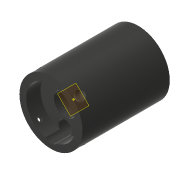
# Autodesk Inventor part: Backshellv1
Saved by Autodesk Inventor 2019.4 (Build 234330000, 330)
## iProperties
Created: 2020-03-14
Part Number: Backshellv1
Material: UHMW, Black
Document SubType Name: Modeling
Designer: Peter
Density: 0.94 g/cm^3
Appearance: Smooth - Black
Mass: 267.904 g
Surface Area: 536.934 cm^2
Volume: 285.004 cm^3
Author: Peter
Autodesk Inventor part; units mm, degrees
ref_plane "YZ Plane" through (0, 0, 0) normal (1, 0, 0) x (0, 1, 0)
ref_plane "XZ Plane" through (0, 0, 0) normal (0, 1, 0) x (-1, 0, 0)
ref_plane "XY Plane" through (0, 0, 0) normal (0, 0, 1) x (1, 0, 0)
sketch "Sketch1" plane through (0, 0, 0) normal (0, 0, 1) x (1, 0, 0)
  circle A0 centre (0, 0) radius 37.5
  dimension "d0" = 75
  constraints: 1 centre point, 1 coincident
  measures "d0" diameter of A0
extrude "Extrusion1" add sketch "Sketch1" along normal blind 104
sketch "Sketch3" plane through (0, 0, 0) normal (0, 0, -1) x (-1, 0, 0)
  circle A0 centre (0, 0) radius 35
  dimension "d6" = 70
  constraints: 1 centre point, 1 coincident
  measures "d6" diameter of A0
extrude "Extrusion3" cut sketch "Sketch3" against normal blind 16.5
sketch "Sketch4" plane through (0, 0, 16.5) normal (0, 0, -1) x (-1, 0, 0)
  circle A0 centre (0, 0) radius 8
  dimension "d9" = 16
  constraints: 1 centre point, 1 coincident
  measures "d9" diameter of A0
extrude "Extrusion4" add sketch "Sketch4" along normal blind 10.5
sketch "Sketch6" plane through (0, 0, 104) normal (0, 0, 1) x (1, 0, 0)
  circle A0 centre (0, 0) radius 16.9805
  constraints: 1 centre point, 1 coincident
hole "Hole1" at (0, 0, 104) direction (0, 0, -1) diameter 27 depth 70 tip angle 118 counterbore diameter 59 counterbore depth 17
sketch "Sketch7" plane through (0, 0, 6) normal (0, 0, -1) x (-1, 0, 0)
  circle A0 centre (0, 0) radius 2.5875
  constraints: 1 centre point, 1 coincident
hole "Hole2" at (0, 0, 6) direction (0, 0, 1) diameter 10.106 end through all thread size "M12x1.75" class "6H" standard "ISO Metric profile"
sketch "Sketch8" plane through (0, 0, 16.5) normal (0, 0, -1) x (-1, 0, 0)
  circle A0 centre (0, 0) radius 24 construction
  circle A1 centre (0, -24) radius 8
  circle A2 centre (0, 24) radius 8
  dimension "d26" = 48
  dimension "d27" = 16
  dimension "d28" = 16
  constraints: 3 centre point, 2 point on circle, 1 coincident
  measures "d26" diameter of A0
  measures "d27" diameter of A2
  measures "d28" diameter of A1
extrude "Extrusion5" cut sketch "Sketch8" against normal through all
sketch "Sketch9" plane through (0, 0, 16.5) normal (0, 0, -1) x (-1, 0, 0)
  circle A0 centre (0, 0) radius 13
  line L0 (0, 0) -> (9.1924, 9.1924)
  line L1 (0, 0) -> (13, 0) construction
  circle A1 centre (9.1924, 9.1924) radius 2.3283
  dimension "d31" = 26
  dimension "d33" = 13
  dimension "d34" = 45
  constraints: 4 end point, 2 centre point, 2 coincident, 1 equal length, 1 horizontal
  measures "d31" diameter of A0
  measures "d33" distance of L0.start L0.end
  measures "d34" angle of L1 L0
hole "Hole3" at (-9.1924, 9.1924, 16.5) direction (0, 0, 1) diameter 6.35 depth 26 tip angle 118
pattern_circular "Circular Pattern1" count 4 over 360 about axis through (0, 0, 154.5463) along (0, 0, -1) of "Hole3"
sketch "Sketch10" plane through (0, 0, 104) normal (0, 0, 1) x (1, 0, 0)
  line L0 (0, 0) -> (26.5165, 26.5165)
  circle A0 centre (0, 0) radius 37.5 projected
  line L1 (0, 0) -> (37.5, 0)
  dimension "d45" = 45
  constraints: 4 end point, 2 point on circle, 1 coincident, 1 horizontal
  measures "d45" angle of L1 L0
ref_plane "Work Plane1" through (26.5165, 26.5165, 104) normal (0.7071, 0.7071, 0) x (-0.7071, 0.7071, 0)
sketch "Sketch11" plane through (26.5165, 26.5165, 104) normal (0.7071, 0.7071, 0) x (-0.7071, 0.7071, 0)
  circle A0 centre (0, -8) radius 3.0843
  line L0 (37.5, 0) -> (-37.5, 0) projected
  point P0 (0, -104)
  dimension "d46" = 8
  constraints: 1 centre point
  measures "d46" distance from line of L0 A0.centre
hole "Hole4" at (26.5165, 26.5165, 96) direction (-0.7071, -0.7071, 0) diameter 5.2 depth 15 tip angle 118 countersink diameter 12 countersink angle 90
pattern_circular "Circular Pattern2" count 4 over 360 about axis through (0, 0, 69) along (0, 0, 1) of "Hole4"
body "Solid1"
